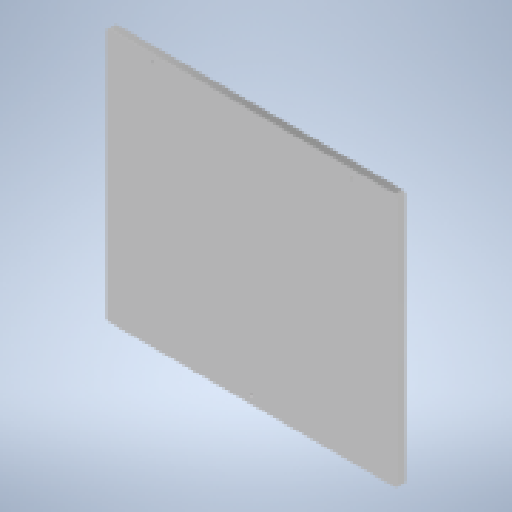
# Autodesk Inventor part: Print Bed R2
Saved by Autodesk Inventor 2024 (Build 280153000, 153)
## iProperties
Created: 2024-12-30
Part Number: Print Bed R2
Material: Aluminum 6061
Document SubType Name: Modeling
Designer: Ishaan
Density: 2.7 g/cm^3
Appearance: Aluminum - Flat
Author: Ishaan
Autodesk Inventor part; units mm, degrees
ref_plane "YZ Plane" through (0, 0, 0) normal (1, 0, 0) x (0, 1, 0)
ref_plane "XZ Plane" through (0, 0, 0) normal (0, 1, 0) x (-1, 0, 0)
ref_plane "XY Plane" through (0, 0, 0) normal (0, 0, 1) x (1, 0, 0)
sketch "Sketch1" plane through (0, 0, 0) normal (0, 0, 1) x (1, 0, 0)
  line L0 (155, -135) -> (-155, -135)
  line L1 (-155, -135) -> (-155, 135)
  line L2 (-155, 135) -> (155, 135)
  line L3 (155, 135) -> (155, -135)
  line L4 (155, -135) -> (-155, 135) construction
  line L5 (-155, -135) -> (155, 135) construction
  line L6 (152.5, -117.5) -> (-152.5, -117.5) construction
  line L7 (-152.5, -117.5) -> (-152.5, 117.5) construction
  line L8 (-152.5, 117.5) -> (152.5, 117.5) construction
  line L9 (152.5, 117.5) -> (152.5, -117.5) construction
  line L10 (152.5, -117.5) -> (-152.5, 117.5) construction
  line L11 (-152.5, -117.5) -> (152.5, 117.5) construction
  circle A0 centre (0, -126.25) radius 8 construction
  circle A1 centre (0, -126.25) radius 4 construction
  line L12 (0, -117.5) -> (0, -135) construction
  line L13 (0, 135) -> (0, 117.5) construction
  line L14 (-105, 126.25) -> (105, 126.25) construction
  circle A2 centre (-105, 126.25) radius 8 construction
  circle A3 centre (105, 126.25) radius 8 construction
  circle A4 centre (105, 126.25) radius 4 construction
  circle A5 centre (-105, 126.25) radius 4 construction
  line L15 (150, -130) -> (-150, -130) construction
  line L16 (-150, -130) -> (-150, 120) construction
  line L17 (-150, 120) -> (150, 120) construction
  line L18 (150, 120) -> (150, -130) construction
  line L19 (150, -130) -> (-150, 120) construction
  line L20 (-150, -130) -> (150, 120) construction
  point P0 (0, 0)
  point P1 (0, -126.25)
  point P2 (0, 126.25)
  point P3 (0, -5)
  dimension "d0" = 310
  dimension "d1" = 270
  dimension "d2" = 305
  dimension "d3" = 235
  dimension "d4" = 16
  dimension "d5" = 8
  dimension "d6" = 210
  dimension "d7" = 300
  dimension "d8" = 250
  dimension "d9" = 5
  dimension "d10" = 5
  constraints: 42 end point, 13 midpoint, 6 centre point, 6 coincident, 6 parallel, 4 equal radius, 4 horizontal, 3 perpendicular
  measures "d0" distance of L1.end L2.end
  measures "d1" distance of L0.end L1.end
  measures "d2" distance of L7.end L8.end
  measures "d3" distance of L6.end L7.end
  measures "d4" diameter of A0
  measures "d5" diameter of A1
  measures "d6" distance of L14.start L14.end
  measures "d7" distance of L16.end L17.end
  measures "d8" distance of L15.end L16.end
  measures "d9" distance between parallel lines of L3 L18
  measures "d10" distance between parallel lines of L0 L15
extrude "Extrusion1" add sketch "Sketch1" along normal blind 7.9375
hole "Hole1" at (0, -126.25, 0) at (105, 126.25, 0) at (-105, 126.25, 0) direction (0, 0, 1) diameter 3.242 end through all thread size "M4x0.7" class "6H" standard "ANSI Metric M Profile"
chamfer "Chamfer3" distance 0.25 angle 45 6 edges at (0, -127.871, 0) (-105, 124.629, 0) (105, 124.629, 0) (0, -127.871, 7.9375) (-105, 124.629, 7.9375) (105, 124.629, 7.9375)
chamfer "Chamfer1" distance 3 angle 45 4 edges at (-155, 135, 3.9688) (155, 135, 3.9688) (155, -135, 3.9688) (-155, -135, 3.9688)
chamfer "Chamfer2" distance 0.25 angle 45 8 edges at (-155, 0, 7.9375) (0, 135, 7.9375) (155, 0, 7.9375) (0, -135, 7.9375) (-155, 0, 0) (0, -135, 0) (155, 0, 0) (0, 135, 0)
equation "\"d10\" = d9"
body "Solid1"
